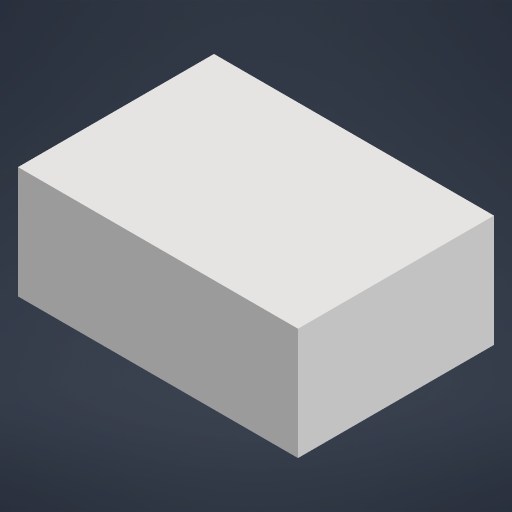
# Autodesk Inventor part: SpinCoater
Saved by Autodesk Inventor 2024.2 (Build 282272000, 272)
## iProperties
Created: 2024-10-04
Part Number: SpinCoater
Material: Generic
Document SubType Name: Modeling
Designer: jerem
Density: 1 g/cm^3
Appearance: Default
Author: jerem
Autodesk Inventor part; units mm, degrees
ref_plane "YZ Plane" through (0, 0, 0) normal (1, 0, 0) x (0, 1, 0)
ref_plane "XZ Plane" through (0, 0, 0) normal (0, 1, 0) x (-1, 0, 0)
ref_plane "XY Plane" through (0, 0, 0) normal (0, 0, 1) x (1, 0, 0)
sketch "Sketch1" plane through (0, 0, 0) normal (0, 1, 0) x (-1, 0, 0)
  line L0 (-125, -87.5) -> (125, -87.5)
  line L1 (125, -87.5) -> (125, 87.5)
  line L2 (125, 87.5) -> (-125, 87.5)
  line L3 (-125, 87.5) -> (-125, -87.5)
  line L4 (-125, -87.5) -> (125, 87.5) construction
  line L5 (125, -87.5) -> (-125, 87.5) construction
  point P0 (0, 0)
  dimension "d0" = 175
  dimension "d1" = 250
  constraints: 12 end point, 2 midpoint, 2 parallel, 1 horizontal, 1 perpendicular
  measures "d0" distance of L0.end L1.end
  measures "d1" distance of L1.end L2.end
extrude "Extrusion1" add sketch "Sketch1" along normal blind 100
body "Solid1"
